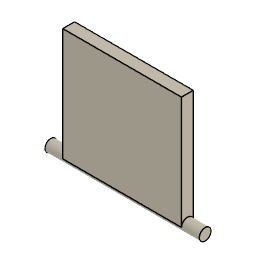
placuta mica (Autodesk Fusion 360 design; units mm, degrees)
part number: 2026-05-04-02-08-36-679
Autodesk Fusion 360 part; units mm, degrees
sketch "Sketch1" plane through (0, 0, 0) normal (0, 1, 0) x (1, 0, 0)
  line L0 (0, 0) -> (0, -19)
  line L1 (0, -19) -> (20, -19)
  line L2 (20, -19) -> (20, 0)
  line L3 (20, 0) -> (0, 0)
  line L4 (0, 0) -> (-3, 0)
  line L5 (-3, 0) -> (-3, 1)
  line L6 (-3, 1) -> (23, 1)
  line L7 (20, 0) -> (23, 0)
  line L8 (23, 0) -> (23, 1)
  dimension "d1" = 19
  dimension "d2" = 20
  dimension "d7" = 3
  dimension "d8" = 3
  dimension "d9" = 1
  constraint coincident L0.start L3.end
  constraint vertical L0
  constraint perpendicular L0 L1
  constraint perpendicular L1 L2
  constraint perpendicular L0 L3
  constraint perpendicular L0 L4
  constraint perpendicular L4 L5
  constraint perpendicular L5 L6
  constraint perpendicular L2 L7
  constraint perpendicular L6 L8
  measures "d1" distance of L0.start L0.end
  measures "d2" distance of L0.end L1.end
  measures "d7" distance of L0 L5
  measures "d8" distance of L2 L8
  measures "d9" distance of L4 L6
revolve "Revolve1" add sketch "Sketch1" angle 360 about axis through (20, 0, 0) along (-1, 0, 0) contours L3 L4 L5 L6 L7 L8
extrude "Extrude1" add sketch "Sketch1" along normal mid plane 2 contours L0 L1 L2 L3
equation "d8 = d7"
